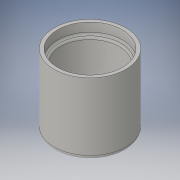
# Autodesk Inventor part: Bolt Cap
Saved by Autodesk Inventor 2016 (Build 200138000, 138)
## iProperties
Created: 2015-07-11
Part Number: Bolt Cap
Material: Generic
Document SubType Name: Modeling
Designer: steele
Density: 1 g/cm^3
Appearance: Default
Author: steele
Autodesk Inventor part; units mm, degrees
ref_plane "YZ Plane" through (0, 0, 0) normal (1, 0, 0) x (0, 1, 0)
ref_plane "XZ Plane" through (0, 0, 0) normal (0, 1, 0) x (-1, 0, 0)
ref_plane "XY Plane" through (0, 0, 0) normal (0, 0, 1) x (1, 0, 0)
sketch "Sketch1" plane through (0, 0, 0) normal (0, 1, 0) x (-1, 0, 0)
  circle A0 centre (0, 0) radius 12.7
  dimension "d1" = 25.4
  constraints: 1 centre point
  measures "d1" diameter of A0
extrude "Extrusion1" add sketch "Sketch1" against normal blind 25.4
shell "Shell1" thickness 2.286 removed faces 1 at (-0.1664, 0, 2.8072)
sketch "Sketch2" plane through (0, 0, 0) normal (0, 1, 0) x (1, 0, 0)
  circle A0 centre (0, 0) radius 11.5189
  dimension "d5" = 23.0378
  constraints: 1 centre point, 1 coincident
  measures "d5" diameter of A0
extrude "Extrusion2" cut sketch "Sketch2" against normal blind 3.81
fillet "Fillet1" radius 1.5875 1 edges at (12.7, -25.4, 0)
fillet "Fillet2" radius 1.5875 1 edges at (10.414, -23.114, 0)
fillet "Fillet3" radius 0.7937 1 edges at (10.414, -3.81, 0)
fillet "Fillet4" radius 0.7937 1 edges at (-11.5189, -3.81, 0)
body "Solid1"
